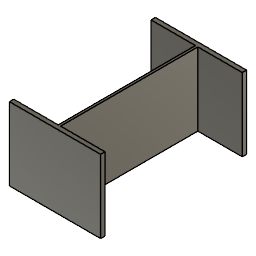
軽H-200×125×3.2×6.0 (Autodesk Fusion 360 design; units mm, degrees)
Autodesk Fusion 360 part; units mm, degrees
sketch "スケッチ1" plane through (0, 0, 0) normal (0, 0, 1) x (1, 0, 0)
  line L0 (62.5, 100) -> (-62.5, 100)
  line L1 (-62.5, -100) -> (62.5, -100)
  line L2 (1.6, 94) -> (1.6, -94)
  line L3 (-1.6, 94) -> (-1.6, -94)
  line L4 (62.5, 94) -> (1.6, 94)
  line L5 (-1.6, 94) -> (-62.5, 94)
  line L6 (-62.5, -94) -> (-1.6, -94)
  line L7 (1.6, -94) -> (62.5, -94)
  line L8 (-62.5, -94) -> (-62.5, -100)
  line L9 (62.5, -94) -> (62.5, -100)
  line L10 (-62.5, 100) -> (-62.5, 94)
  line L11 (62.5, 100) -> (62.5, 94)
  dimension "d1" = 125
  dimension "d2" = 200
  constraint horizontal L0
  constraint parallel L0 L1
  constraint coincident L3.start L4
  constraint collinear L4 L5
  constraint collinear L6 L7
  constraint perpendicular L6 L8
  constraint perpendicular L1 L9
  constraint perpendicular L5 L10
  constraint perpendicular L4 L11
  measures "d1" distance of L1.start L1.end
  measures "d2" distance of L0.end L1.start
extrude "押し出し1" add sketch "スケッチ1" along normal blind 100
